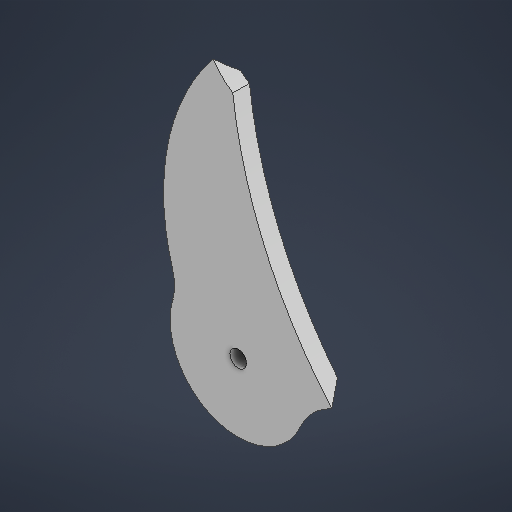
# Autodesk Inventor part: Hoja de Corte
Saved by Autodesk Inventor 2026.1 (Build 301233020, 233B)
## iProperties
Created: 2025-11-03
Part Number: Hoja de Corte
Material: Generic
Document SubType Name: Modeling
Designer: Marcelo
Density: 1 g/cm^3
Appearance: Default
Author: Marcelo
Autodesk Inventor part; units mm, degrees
note: some values were not read from the file. Chosen so that the rebuilt part matches the saved one: second side of "Extrusion2".
ref_plane "YZ Plane" through (0, 0, 0) normal (1, 0, 0) x (0, 1, 0)
ref_plane "XZ Plane" through (0, 0, 0) normal (0, 1, 0) x (-1, 0, 0)
ref_plane "XY Plane" through (0, 0, 0) normal (0, 0, 1) x (1, 0, 0)
sketch "Sketch1" plane through (0, 0, 0) normal (0, 0, 1) x (1, 0, 0)
  arc A0 (-12.435485, 76.169317) -> (-19.719816, 39.609757) centre (18.622974, 50.975591) ccw
  arc A1 (-12.435485, 76.169317) -> (-8.899951, 72.633783) centre (-2.589145, 82.480123) ccw
  line L0 (-12.435485, 76.169317) -> (-8.899951, 72.633783) construction
  line L1 (-12.435485, 76.169317) -> (-7.435485, 76.169317) construction
  arc A2 (-8.899951, 72.633783) -> (8.917299, 32.302519) centre (65.581671, 81.436509) ccw
  arc A3 (8.917299, 32.302519) -> (3.260445, 26.645665) centre (13.582916, 21.980048) ccw
  line L2 (8.917299, 32.302519) -> (3.260445, 26.645665) construction
  line L3 (8.917299, 32.302519) -> (16.917299, 32.302519) construction
  arc A4 (-19.70552, 35.111295) -> (3.260445, 26.645665) centre (-7.920046, 31.699095) ccw
  arc A5 (-19.70552, 35.111295) -> (-19.719816, 39.609757) centre (-27.389927, 37.336129) ccw
  circle A6 centre (-7.920046, 31.699095) radius 1.5
  line L4 (-21.368921, 76.169317) -> (8.917299, 76.169317)
  line L5 (8.917299, 76.169317) -> (8.917299, 19.429599)
  line L6 (8.917299, 19.429599) -> (-21.368921, 19.429599)
  line L7 (-21.368921, 19.429599) -> (-21.368921, 76.169317)
  line L8 (-21.368921, 39.609757) -> (3.327974, 39.609757)
  line L9 (-19.719816, 39.609757) -> (3.327974, 39.609757) construction
  line L10 (3.327974, 39.609757) -> (3.327974, 76.169317)
  line L11 (3.327974, 39.609757) -> (39.887534, 39.609757) construction
  dimension "d25" = 39.9919
  dimension "d26" = 5
  dimension "d27" = 45
  dimension "d28" = 75
  dimension "d29" = 8
  dimension "d30" = 135
  dimension "d31" = 8
  dimension "d32" = 3
  dimension "d51" = 0
  dimension "d52" = 90
  constraints: 24 end point, 13 point on circle, 7 centre point, 5 horizontal, 5 point on line, 5 tangent, 3 equal length, 2 parallel, 1 coincident, 1 perpendicular
  measures "d25" radius of A0
  measures "d26" distance of L0.start L0.end
  measures "d27" angle of L0 L1
  measures "d28" radius of A2
  measures "d29" distance of L2.start L2.end
  measures "d30" angle of L2 L3
  measures "d31" radius of A5
  measures "d32" diameter of A6
  measures "d51" distance between parallel lines of L8 L9
  measures "d52" angle of L11 L10
sketch "Sketch1 outline for Extrusion1" plane through (0, 0, 0) normal (0, 0, 1) x (1, 0, 0)
  arc A0 (-8.899951, 72.633783) -> (-12.435485, 76.169317) centre (-2.589145, 82.480123) cw
  arc A1 (8.917299, 32.302519) -> (-8.899951, 72.633783) centre (65.581671, 81.436509) cw
  arc A2 (-12.435485, 76.169317) -> (-19.719816, 39.609757) centre (18.622974, 50.975591) ccw
  arc A3 (3.260445, 26.645665) -> (8.917299, 32.302519) centre (13.582916, 21.980048) cw
  arc A4 (-19.719816, 39.609757) -> (-19.70552, 35.111295) centre (-27.389927, 37.336129) cw
  arc A5 (-19.70552, 35.111295) -> (3.260445, 26.645665) centre (-7.920046, 31.699095) ccw
  circle A6 centre (-7.920046, 31.699095) radius 1.5
extrude "Extrusion1" add sketch "Sketch1 outline for Extrusion1" along normal blind 3
sketch "Sketch2" plane through (0, 0, 0) normal (0, 0, -1) x (-1, 0, 0)
  arc A0 (8.899951, 72.633783) -> (12.435485, 76.169317) centre (2.589145, 82.480123) ccw
  arc A1 (19.719816, 39.609757) -> (12.435485, 76.169317) centre (-18.622974, 50.975591) ccw
  arc A2 (-8.917299, 32.302519) -> (8.899951, 72.633783) centre (-65.581671, 81.436509) ccw
  arc A3 (19.719816, 39.609757) -> (19.70552, 35.111295) centre (27.389927, 37.336129) ccw
  line L0 (19.719816, 39.609757) -> (0.192482, 45.398184)
  arc A4 (11.216243, 74.583931) -> (12.435485, 76.169317) centre (2.589145, 82.480123) ccw
  arc A5 (9.327537, 42.690308) -> (11.216243, 74.583931) centre (-26.326768, 60.804454) ccw
  point P0 (0, 0)
  dimension "d35" = 0
  dimension "d37" = 2
  constraints: 6 point on circle, 2 centre point, 2 end point, 2 equal radius, 1 point on line
  measures "d35" distance from line of A1.centre L0
  measures "d37" distance of A0.end A4.start
sketch "Sketch2 outline for Extrusion2" plane through (0, 0, 0) normal (0, 0, -1) x (-1, 0, 0)
  arc A0 (19.719816, 39.609757) -> (12.435485, 76.169317) centre (-18.622974, 50.975591) ccw
  line L0 (9.327537, 42.690308) -> (19.719816, 39.609757)
  arc A1 (11.216243, 74.583931) -> (9.327537, 42.690308) centre (-26.326768, 60.804454) cw
  arc A2 (12.435485, 76.169317) -> (11.216243, 74.583931) centre (2.589145, 82.480123) cw
extrude "Extrusion2" add sketch "Sketch2 outline for Extrusion2" against normal blind 3
sketch "Sketch5" plane through (0, 0, 3) normal (0, 0, 1) x (1, 0, 0)
  line L0 (-9.327537, 42.690308) -> (-19.719816, 39.609757)
  line L1 (-9.327537, 42.690308) -> (-9.327537, 72.921318)
  arc A0 (-12.435485, 76.169317) -> (-8.899951, 72.633783) centre (-2.589145, 82.480123) ccw
  line L2 (-9.327537, 42.690308) -> (20.903473, 42.690308) construction
  line L3 (-19.719816, 39.609757) -> (-9.327537, 39.609757)
  line L4 (-19.719816, 39.609757) -> (-9.327537, 39.609757) construction
  line L5 (-9.327537, 39.609757) -> (-9.327537, 42.690308)
  line L6 (-21.368921, 76.169317) -> (-21.368921, 42.690308)
  arc A1 (-12.435485, 76.169317) -> (-19.719816, 39.609757) centre (18.622974, 50.975591) ccw
  line L7 (-19.719816, 39.609757) -> (-21.368921, 39.609757)
  line L8 (-21.368921, 39.609757) -> (-21.368921, 43.268072)
  line L9 (-21.368921, 76.169317) -> (-9.327537, 76.169317)
  line L10 (-9.327537, 72.921318) -> (-9.327537, 76.169317)
  point P0 (0, 0)
  point P1 (-11.216243, 74.583931)
  point P2 (-21.368921, 50.975591)
  dimension "d47" = 90
  dimension "d48" = 0
  constraints: 20 end point, 5 point on line, 3 horizontal, 2 equal length, 2 point on circle, 2 vertical, 1 perpendicular, 1 tangent
  measures "d47" angle of L2 L1
  measures "d48" distance between parallel lines of L3 L4
sketch "Sketch6" plane through (0, 0, 3) normal (0, 0, 1) x (-1, 0, 0)
  line L0 (21.368921, -76.169317) -> (21.368921, -42.690308)
  arc A0 (19.719816, 39.609757) -> (12.435485, 76.169317) centre (-18.622974, 50.975591) ccw
  point P0 (0, 0)
  point P1 (21.368921, 50.975591)
  constraints: 1 point on circle, 1 point on line
ref_plane "Work Plane3" through (-9.327537, 76.169317, 3) normal (0, 0, -1) x (0, -1, 0)
extrude "Extrusion3" [suppressed]
draft "FaceDraft7" angle 45 pull direction (0, 0, -1) faces at (-13.99815, 74.110283, 1) (-19.580116, 35.602105, 2) (0.992604, 23.266705, 2) (3.667398, 27.457629, 1) fixed edges at (-20.597986, 58.790194, 3) (-19.389968, 37.361551, 3) (-12.163655, 20.186828, 3) (5.572879, 29.990085, 3)
body "Solid1"
